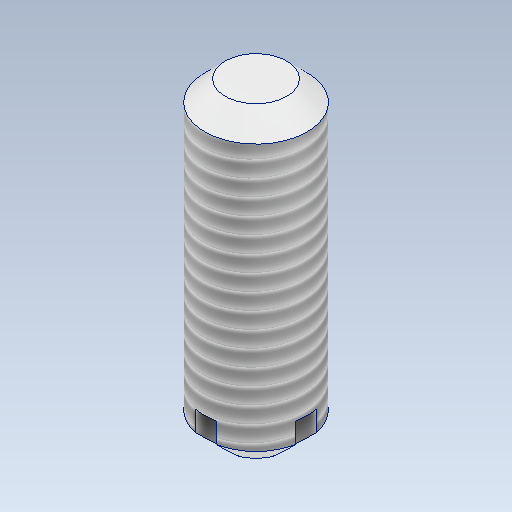
# Autodesk Inventor part: M5x15
Saved by Autodesk Inventor 2020 (Build 240168000, 168)
## iProperties
Created: 2021-03-23
Part Number: M5x15
Material: Aluminum 6061
Document SubType Name: Modeling
Designer: patry
Density: 2.7 g/cm^3
Appearance: Aluminum - Flat
Mass: 0.715672 g
Surface Area: 2.75257 cm^2
Volume: 0.265064 cm^3
Author: patry
Autodesk Inventor part; units mm, degrees
ref_plane "YZ Plane" through (0, 0, 0) normal (1, 0, 0) x (0, 1, 0)
ref_plane "XZ Plane" through (0, 0, 0) normal (0, 1, 0) x (-1, 0, 0)
ref_plane "XY Plane" through (0, 0, 0) normal (0, 0, 1) x (1, 0, 0)
sketch "Szkic1" plane through (0, 0, 0) normal (0, 1, 0) x (-1, 0, 0)
  circle A0 centre (0, 0) radius 4.25
  line L0 (1.1547, 2) -> (2.3094, 0)
  line L1 (2.3094, 0) -> (1.1547, -2)
  line L2 (1.1547, -2) -> (-1.1547, -2)
  line L3 (-1.1547, -2) -> (-2.3094, 0)
  line L4 (-2.3094, 0) -> (-1.1547, 2)
  line L5 (-1.1547, 2) -> (1.1547, 2)
  circle A1 centre (0, 0) radius 2.5
  dimension "d0" = 8.5
  dimension "d1" = 4
  dimension "d2" = 5
  constraints: 12 end point, 3 coincident, 2 centre point, 13 other
  measures "d0" diameter of A0
  measures "d1" distance between parallel lines of L2 L5
  measures "d2" diameter of A1
extrude "Wyciągnięcie proste4" add sketch "Szkic1" along normal blind 15 contours L0 L1 L2 L3 L4 L5 | A1
thread "Gwint2" size "M5x0.8" class "6g" standard "ANSI Metric M Profile" full length
chamfer "Faza1" distance 1 angle 45 1 edges at (2.5, 15, 0)
chamfer "Faza2" distance 1 angle 45 1 edges at (2.5, 0, 0)
sketch "Szkic3" plane through (0, 0, 0) normal (0, -1, 0) x (1, 0, 0)
  circle A0 centre (0, 0) radius 2.5 projected
  line L0 (2.5, 0) -> (-2.5, 0) construction
  line L1 (0, 2.5) -> (0, 0.5) construction
  line L2 (0.5, 2.5) -> (0.5, 2.4495) construction
  line L3 (-0.5, 2.5) -> (-0.5, 2.4495) construction
  line L4 (2.5, 0.5) -> (2.4495, 0.5) construction
  line L5 (2.5, -0.5) -> (2.4495, -0.5) construction
  circle A1 centre (0, 0) radius 2.5 construction
  line L6 (2.4495, 0.5) -> (0.5, 0.5)
  line L7 (2.4495, -0.5) -> (0.5, -0.5)
  line L8 (0.5, 2.4495) -> (0.5, 0.5)
  line L9 (-0.5, 2.4495) -> (-0.5, 0.5)
  line L10 (-0.5, 0.5) -> (-0.5, -0.5) construction
  line L11 (0.5, 0.5) -> (0.5, -0.5) construction
  line L12 (0.5, -0.5) -> (-0.5, -0.5) construction
  line L13 (-0.5, -0.5) -> (-0.5, -2.4495)
  line L14 (-2.4495, -0.5) -> (-2.5, -0.5) construction
  line L15 (-2.4495, 0.5) -> (-2.5, 0.5) construction
  line L16 (-0.5, -2.4495) -> (-0.5, -2.5) construction
  line L17 (0.5, -2.4495) -> (0.5, -2.5) construction
  line L18 (0.5, -0.5) -> (0.5, -2.4495)
  line L19 (0.5, 0.5) -> (-0.5, 0.5) construction
  line L20 (0, 0.5) -> (0, -2.5) construction
  line L21 (-0.5, -0.5) -> (-2.4495, -0.5)
  line L22 (-0.5, 0.5) -> (-2.4495, 0.5)
  dimension "d22" = 0.5
  dimension "d23" = 0.5
  dimension "d24" = 0.5
  dimension "d25" = 0.5
  constraints: 46 end point, 30 parallel, 4 point on circle, 2 perpendicular, 1 horizontal, 1 midpoint, 1 point on line, 9 other
  measures "d22" distance between parallel lines of L1 L2
  measures "d23" distance between parallel lines of L1 L3
  measures "d24" distance between parallel lines of L0 L4
  measures "d25" distance between parallel lines of L0 L5
extrude "Wyciągnięcie proste5" cut sketch "Szkic3" against normal blind 2 contours A0 L7 L18 L13 L21 L22 L9 L8 L6
